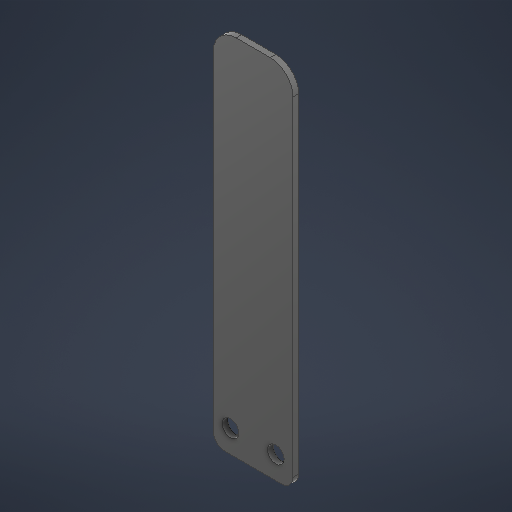
# Autodesk Inventor part: American Flag Replacement
Saved by Autodesk Inventor 2025 (Build 290162000, 162)
## iProperties
Created: 2024-12-29
Part Number: American Flag Replacement
Material: Generic
Document SubType Name: Modeling
Designer: Juan
Density: 1 g/cm^3
Appearance: Default
Author: Juan
Autodesk Inventor part; units mm, degrees
ref_plane "YZ Plane" through (0, 0, 0) normal (1, 0, 0) x (0, 1, 0)
ref_plane "XZ Plane" through (0, 0, 0) normal (0, 1, 0) x (-1, 0, 0)
ref_plane "XY Plane" through (0, 0, 0) normal (0, 0, 1) x (1, 0, 0)
sketch "Sketch1" plane through (0, 0, 0) normal (0, 0, 1) x (1, 0, 0)
  circle A0 centre (0, 0) radius 2.3241
  line L0 (0, 0) -> (12.7, 0)
  line L1 (0, 0) -> (-12.7, 0)
  circle A1 centre (-12.7, 0) radius 2.3241
  circle A2 centre (12.7, 0) radius 2.3241
  line L2 (-19.05, -6.35) -> (19.05, -6.35)
  line L3 (19.05, -6.35) -> (19.05, 6.35)
  line L4 (19.05, 6.35) -> (-19.05, 6.35)
  line L5 (-19.05, 6.35) -> (-19.05, -6.35)
  line L6 (-19.05, -6.35) -> (19.05, 6.35) construction
  line L7 (19.05, -6.35) -> (-19.05, 6.35) construction
  line L8 (-19.05, 6.35) -> (19.05, 6.35)
  line L9 (19.05, 6.35) -> (19.05, 95.25)
  line L10 (19.05, 95.25) -> (-19.05, 95.25)
  line L11 (-19.05, 95.25) -> (-19.05, 6.35)
  line L12 (-19.05, -6.35) -> (-17.4625, -6.35)
  line L13 (19.05, -6.35) -> (17.4625, -6.35)
  line L14 (-17.4625, -6.35) -> (-17.4625, 95.25)
  line L15 (17.4625, -6.35) -> (17.4625, 95.25)
  dimension "d0" = 4.6482
  dimension "d1" = 12.7
  dimension "d2" = 12.7
  dimension "d3" = 4.6482
  dimension "d4" = 4.6482
  dimension "d5" = 38.1
  dimension "d6" = 12.7
  dimension "d7" = 88.9
  dimension "d8" = 38.1
  dimension "d11" = 1.5875
  dimension "d12" = 1.5875
  constraints: 32 end point, 4 parallel, 4 perpendicular, 4 point on line, 3 centre point, 3 coincident, 3 horizontal, 2 midpoint
  measures "d0" diameter of A0
  measures "d1" distance of L0.start L0.end
  measures "d2" distance of L0.start L1.end
  measures "d3" diameter of A1
  measures "d4" diameter of A2
  measures "d5" distance of L2.start L2.end
  measures "d6" distance of L3.end L2.end
  measures "d7" distance of L8.end L9.end
  measures "d8" distance of L9.end L10.end
  measures "d11" distance of L2.start L12.end
  measures "d12" distance of L2.end L13.end
extrude "Extrusion1" add sketch "Sketch1" along normal blind 1.5875
extrude "Extrusion2" cut sketch "Sketch1" along normal through all contours L5 L4 L14 L2 | L11 L10 L14 L4 | L15 L4 L3 L2 | L15 L10 L9 L4
fillet "Fillet1" radius 3.175 2 edges at (-17.4625, -6.35, 0.7937) (17.4625, -6.35, 0.7937)
fillet "Fillet2" radius 6.35 2 edges at (-17.4625, 95.25, 0.7937) (17.4625, 95.25, 0.7937)
sketch "Sketch2" plane through (0, 0, 1.5875) normal (0, 0, 1) x (1, 0, 0)
  arc A0 (17.4625, 88.9) -> (11.1125, 95.25) centre (11.1125, 88.9) ccw projected
  line L0 (11.1125, 95.25) -> (-11.1125, 95.25) projected
  arc A1 (-11.1125, 95.25) -> (-17.4625, 88.9) centre (-11.1125, 88.9) ccw projected
  line L1 (-17.4625, 88.9) -> (-17.4625, -3.175) projected
  arc A2 (-17.4625, -3.175) -> (-14.2875, -6.35) centre (-14.2875, -3.175) ccw projected
  line L2 (-14.2875, -6.35) -> (14.2875, -6.35) projected
  arc A3 (14.2875, -6.35) -> (17.4625, -3.175) centre (14.2875, -3.175) ccw projected
  line L3 (17.4625, -3.175) -> (17.4625, 88.9) projected
  circle A4 centre (12.7, 0) radius 2.3241 projected
  circle A5 centre (0, 0) radius 2.3241 projected
  circle A6 centre (-12.7, 0) radius 2.3241 projected
  line L4 (-17.4625, 10.0615) -> (-4.7625, 10.0615)
  line L5 (-4.7625, -6.35) -> (-31.8174, -6.35)
  line L6 (-31.8174, -6.35) -> (-31.8174, 101.6265)
  line L7 (-31.8174, 101.6265) -> (-4.7625, 101.6265)
  line L8 (-4.7625, 101.6265) -> (-4.7625, -6.35)
  point P0 (-4.7625, 95.25)
  dimension "d17" = 12.7
  constraints: 10 end point, 2 horizontal, 2 parallel, 2 point on line, 1 perpendicular
  measures "d17" distance of L4.start L4.end
extrude "Extrusion3" cut sketch "Sketch2" against normal blind 25.4 contours L8 L4 L1 A1 L0 | L8 L2 A2 L1 L4
fillet "Fillet3" radius 3.175 1 edges at (-4.7625, -6.35, 0.7937)
fillet "Fillet4" radius 6.35 1 edges at (-4.7625, 95.25, 0.7937)
body "Solid1"
